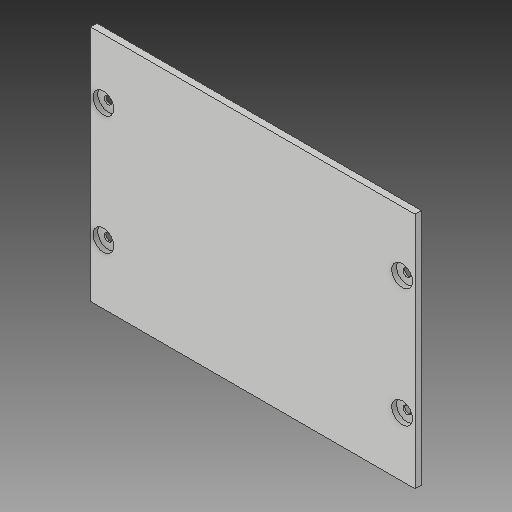
# Autodesk Inventor part: Ra-Manager_Painel-Placas_Tras_Plugs
Saved by Autodesk Inventor 2019.4 (Build 234330000, 330)
## iProperties
Created: 2020-03-24
Part Number: Ra-Manager_Painel-Placas_Tras_Plugs
Material: Genérico
Document SubType Name: Modeling
Designer: caiom
Density: 1 g/cm^3
Appearance: Padrão
Author: caiom
Autodesk Inventor part; units mm, degrees
ref_plane "YZ Plane" through (0, 0, 0) normal (1, 0, 0) x (0, 1, 0)
ref_plane "XZ Plane" through (0, 0, 0) normal (0, 1, 0) x (-1, 0, 0)
ref_plane "XY Plane" through (0, 0, 0) normal (0, 0, 1) x (1, 0, 0)
sketch "Esboço1" plane through (0, 0, 0) normal (0, 0, 1) x (1, 0, 0)
  line L0 (-50.5, -37) -> (50.5, -37)
  line L1 (50.5, -37) -> (50.5, 37)
  line L2 (50.5, 37) -> (-50.5, 37)
  line L3 (-50.5, 37) -> (-50.5, -37)
  point P0 (0, 0)
  point P1 (0, 0)
  dimension "d17" = 101
  dimension "d18" = 74
  dimension "d19" = 50.5
  dimension "d20" = 37
  dimension "d21" = 50.5
  dimension "d22" = 37
  constraints: 8 end point, 2 parallel, 1 perpendicular, 1 vertical
  measures "d17" distance between parallel lines of L1 L3
  measures "d18" distance between parallel lines of L0 L2
  measures "d19" distance from line of point (0, 0) L1
  measures "d20" distance from line of point (0, 0) L2
  measures "d21" distance from line of point (0, 0) L1
  measures "d22" distance from line of point (0, 0) L2
extrude "Extrusão1" add sketch "Esboço1" against normal blind 2
sketch "Esboço2" plane through (0, 0, 0) normal (0, 0, 1) x (1, 0, 0)
  line L0 (-50.5, -37) -> (-50.5, 37)
  line L1 (-50.5, 37) -> (50.5, 37)
  line L2 (-46.5, 37) -> (-46.5, -37) construction
  line L3 (50.5, -37) -> (-50.5, -37)
  line L4 (46.5, 37) -> (46.5, -37) construction
  line L5 (-50.5, 18.5) -> (50.5, 18.5) construction
  line L6 (-50.5, -18.5) -> (50.5, -18.5) construction
  line L7 (50.5, 37) -> (50.5, -37)
  point P0 (0, 0)
  point P1 (0, 0)
  point P2 (-46.5, 18.5)
  point P3 (-46.5, -18.5)
  point P4 (46.5, -18.5)
  point P5 (46.5, 18.5)
  dimension "d28" = 4
  dimension "d29" = 97
  dimension "d30" = 101
  dimension "d31" = 55.5
  dimension "d32" = 18.5
  dimension "d33" = 74
  dimension "d34" = 50.5
  dimension "d35" = 37
  dimension "d36" = 0
  constraints: 16 end point, 15 point on line, 5 parallel, 2 horizontal, 1 perpendicular
  measures "d28" distance between parallel lines of L7 L4
  measures "d29" distance between parallel lines of L7 L2
  measures "d30" distance between parallel lines of L7 L0
  measures "d31" distance between parallel lines of L5 L3
  measures "d32" distance between parallel lines of L6 L3
  measures "d33" distance between parallel lines of L1 L3
  measures "d34" distance from line of point (0, 0) L7
  measures "d35" distance from line of point (0, 0) L3
  measures "d36" distance from line of L5.end L7
hole "Furo1" at (-46.5, 18.5, 0) at (-46.5, -18.5, 0) at (46.5, -18.5, 0) at (46.5, 18.5, 0) direction (0, 0, -1) diameter 2.459 end through all counterbore diameter 6.5 counterbore depth 1.5
